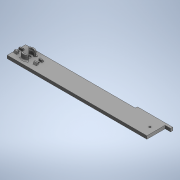
# Autodesk Inventor part: Arm Bottom Left
Saved by Autodesk Inventor 2020.5 (Build 245400000, 400)
## iProperties
Created: 2023-03-21
Part Number: Arm Bottom Left
Material: Generic
Document SubType Name: Modeling
Designer: Wes
Density: 1 g/cm^3
Appearance: Default
Author: Wes
Autodesk Inventor part; units mm, degrees
ref_plane "YZ Plane" through (0, 0, 0) normal (1, 0, 0) x (0, 1, 0)
ref_plane "XZ Plane" through (0, 0, 0) normal (0, 1, 0) x (-1, 0, 0)
ref_plane "XY Plane" through (0, 0, 0) normal (0, 0, 1) x (1, 0, 0)
sketch "Base" plane through (0, 0, 0) normal (0, 0, 1) x (1, 0, 0)
  line L0 (0, 0) -> (-30, 0)
  line L1 (-30, 0) -> (-30, 230)
  line L2 (-30, 230) -> (0, 230)
  line L3 (0, 230) -> (0, 0)
  dimension "d0" = 30
  dimension "d1" = 230
  constraints: 8 end point, 2 parallel, 1 horizontal, 1 perpendicular
  measures "d0" distance of L1.end L2.end
  measures "d1" distance of L0.end L1.end
extrude "Extrusion1" add sketch "Base" along normal blind 5
sketch "Axle Screw Countersink" plane through (0, 0, 5) normal (0, 0, 1) x (1, 0, 0)
  line L0 (-15, 0) -> (-15, 20) construction
  circle A0 centre (-15, 20) radius 3.15
  dimension "d4" = 20
  dimension "d58" = 6.3
  constraints: 2 end point, 1 centre point, 1 coincident, 1 vertical
  measures "d4" distance of L0.start L0.end
  measures "d58" diameter of A0
extrude "Extrusion2" cut sketch "Axle Screw Countersink" against normal blind 1.2
sketch "Motor Arm Center Fitting" plane through (0, 0, 5) normal (0, 0, 1) x (1, 0, 0)
  line L0 (-19.393, 15.95) -> (-19.393, 24.05) construction
  arc A0 (-19.393, 24.05) -> (-19.393, 15.95) centre (-15, 20) ccw
  line L1 (-19.393, 15.95) -> (-21.231, 14.2554)
  line L2 (-19.393, 24.05) -> (-21.231, 25.7446)
  line L3 (-15, 8.3504) -> (-15, 30.6989) construction
  arc A1 (-21.231, 25.7446) -> (-21.231, 14.2554) centre (-15, 20) ccw
  line L4 (-10.607, 15.95) -> (-10.607, 24.05) construction
  line L5 (-10.607, 15.95) -> (-19.393, 15.95) construction
  arc A2 (-10.607, 15.95) -> (-10.607, 24.05) centre (-15, 20) ccw
  line L6 (-10.607, 15.95) -> (-8.769, 14.2554)
  line L7 (-10.607, 24.05) -> (-8.769, 25.7446)
  arc A3 (-8.769, 14.2554) -> (-8.769, 25.7446) centre (-15, 20) ccw
  circle A4 centre (-15, 20) radius 5.975 construction
  point P0 (0, 0)
  point P1 (-15, 20)
  dimension "d18" = 11.95
  dimension "d19" = 8.1
  dimension "d20" = 8.1
  dimension "d21" = 2.5
  dimension "d22" = 2.5
  constraints: 16 end point, 12 point on circle, 5 centre point, 2 line through centre, 2 symmetric about line, 2 vertical, 1 concentric, 1 perpendicular, 2 other
  measures "d18" diameter of A4
  measures "d19" distance of L5.start L4.end
  measures "d20" distance of L5.end L0.end
  measures "d21" distance of L5.end L1.end
  measures "d22" distance of L0.end L2.end
extrude "Extrusion3" add sketch "Motor Arm Center Fitting" along normal blind 5
sketch "Motor Rotation Support" plane through (0, 0, 10) normal (0, 0, 1) x (1, 0, 0)
  line L0 (-20.975, 20) -> (-21.775, 20) construction
  circle A0 centre (-15, 20) radius 6.775 construction
  arc A1 (-19.9811, 24.5923) -> (-19.9811, 15.4077) centre (-15, 20) ccw
  line L1 (-21.775, 20) -> (-23.775, 20) construction
  circle A2 centre (-15, 20) radius 8.775 construction
  arc A3 (-21.4516, 25.9479) -> (-21.4516, 14.0521) centre (-15, 20) ccw
  line L2 (-21.4516, 14.0521) -> (-19.9811, 15.4077)
  line L3 (-19.9811, 24.5923) -> (-21.4516, 25.9479)
  line L4 (-15, 8.5295) -> (-15, 32.0479) construction
  line L5 (-8.5484, 14.0521) -> (-10.0189, 15.4077)
  arc A4 (-8.5484, 14.0521) -> (-8.5484, 25.9479) centre (-15, 20) ccw
  arc A5 (-10.0189, 15.4077) -> (-10.0189, 24.5923) centre (-15, 20) ccw
  line L6 (-10.0189, 24.5923) -> (-8.5484, 25.9479)
  point P0 (0, 0)
  point P1 (-21.231, 14.2554)
  point P2 (-21.231, 25.7446)
  dimension "d25" = 0.8
  dimension "d26" = 2
  constraints: 16 point on circle, 14 end point, 6 centre point, 4 symmetric about line, 2 coincident, 2 horizontal, 1 concentric, 1 vertical, 2 other
  measures "d25" distance of L0.start L0.end
  measures "d26" distance of L0.end L1.end
extrude "Extrusion4" add sketch "Motor Rotation Support" along normal blind 3.35
sketch "Motor Arm Screw Holes" plane through (0, 0, 5) normal (0, 0, 1) x (1, 0, 0)
  line L0 (-15, 20) -> (-15, 37.1) construction
  line L1 (-15, 20) -> (-15, 2.9) construction
  line L2 (-15, 20) -> (-15, 4.2) construction
  line L3 (-15, 20) -> (-15, 35.8) construction
  line L4 (-15, 4.2) -> (-15, 2.9) construction
  line L5 (-15, 35.8) -> (-15, 37.1) construction
  circle A0 centre (-15, 36.45) radius 1.175
  circle A1 centre (-15, 3.55) radius 1.175
  point P0 (0, 0)
  dimension "d59" = 34.2
  dimension "d60" = 31.6
  dimension "d61" = 2.35
  dimension "d62" = 2.35
  constraints: 12 end point, 3 vertical, 2 centre point, 2 midpoint, 2 point on line, 1 coincident, 1 collinear
  measures "d59" distance of L0.end L1.end
  measures "d60" distance of L3.end L2.end
  measures "d61" diameter of A0
  measures "d62" diameter of A1
extrude "Extrusion5" cut sketch "Motor Arm Screw Holes" against normal through all
sketch "Motor Arm Support" plane through (0, 0, 5) normal (0, 0, 1) x (1, 0, 0)
  line L0 (-15, 2.375) -> (-15, 6.875) construction
  line L1 (-15, 6.875) -> (-11.875, 6.875) construction
  line L2 (-15, 6.875) -> (-18.125, 6.875) construction
  line L3 (-21.0644, 20.2154) -> (-9.1144, 20.2154) construction
  line L4 (-15, 3.55) -> (-12.2, 3.55) construction
  line L5 (-15, 3.55) -> (-12.2, 3.55) construction
  line L6 (-15, 3.55) -> (-17.8, 3.55) construction
  line L7 (-15, 3.55) -> (-12.2, 3.55) construction
  line L8 (-18.125, 6.875) -> (-17.8, 3.55)
  line L9 (-17.8, 3.55) -> (-19.7905, 3.3554)
  line L10 (-19.7905, 3.3554) -> (-20.1155, 6.6804)
  line L11 (-20.1155, 6.6804) -> (-18.125, 6.875)
  line L12 (-11.875, 6.875) -> (-12.2, 3.55)
  line L13 (-12.2, 3.55) -> (-10.2095, 3.3554)
  line L14 (-9.8845, 6.6804) -> (-11.875, 6.875)
  line L15 (-10.2095, 3.3554) -> (-9.8845, 6.6804)
  line L16 (-17.8, 3.55) -> (-17.6054, 1.5595)
  line L17 (-17.6054, 1.5595) -> (-19.596, 1.3649)
  line L18 (-19.596, 1.3649) -> (-19.7905, 3.3554)
  line L19 (-12.2, 3.55) -> (-12.3946, 1.5595)
  line L20 (-12.3946, 1.5595) -> (-10.404, 1.3649)
  line L21 (-10.404, 1.3649) -> (-10.2095, 3.3554)
  line L22 (-17.8, 36.8809) -> (-19.7905, 37.0755)
  line L23 (-17.8, 36.8809) -> (-17.6054, 38.8714)
  line L24 (-17.6054, 38.8714) -> (-19.596, 39.066)
  line L25 (-19.596, 39.066) -> (-19.7905, 37.0755)
  line L26 (-18.125, 33.5559) -> (-17.8, 36.8809)
  line L27 (-19.7905, 37.0755) -> (-20.1155, 33.7505)
  line L28 (-20.1155, 33.7505) -> (-18.125, 33.5559)
  line L29 (-11.875, 33.5559) -> (-12.2, 36.8809)
  line L30 (-12.3946, 38.8714) -> (-10.404, 39.066)
  line L31 (-12.2, 36.8809) -> (-10.2095, 37.0755)
  line L32 (-10.404, 39.066) -> (-10.2095, 37.0755)
  line L33 (-10.2095, 37.0755) -> (-9.8845, 33.7505)
  line L34 (-9.8845, 33.7505) -> (-11.875, 33.5559)
  line L35 (-12.2, 36.8809) -> (-12.3946, 38.8714)
  point P0 (0, 0)
  dimension "d63" = 4.5
  dimension "d64" = 6.25
  dimension "d65" = 5.6
  dimension "d66" = 2
  dimension "d67" = 2
  constraints: 72 end point, 18 symmetric about line, 7 horizontal, 5 perpendicular, 2 collinear, 1 vertical
  measures "d63" distance of L0.start L1.start
  measures "d64" distance of L2.end L1.end
  measures "d65" distance of L8.end L4.end
  measures "d66" distance of L8.end L10.start
  measures "d67" distance of L8.end L17.start
extrude "Extrusion6" add sketch "Motor Arm Support" along normal blind 3
draft "FaceDraft1" angle 28 pull direction (0, 0, 1) faces at (-10.2309, 3.1368, 6) (-10.0577, 35.5223, 6) fixed edges at (-10.1443, 4.0227, 8) (-10.1443, 36.4082, 8)
draft "FaceDraft2" angle 28 pull direction (0, 0, 1) faces at (-19.7691, 37.2941, 6) (-19.9423, 4.9086, 6) fixed edges at (-19.8557, 36.4082, 8) (-19.8557, 4.0227, 8)
fillet "Fillet1" radius 2 4 edges at (-23.475, 20, 5) (-6.525, 20, 5) (-8.225, 20, 10) (-21.775, 20, 10)
sketch "Axle Hole" plane through (0, 0, 5) normal (0, 0, 1) x (1, 0, 0)
  line L0 (0, 230) -> (-30, 230) construction
  line L1 (-15, 230) -> (-15, 220) construction
  circle A0 centre (-15, 220) radius 1.5
  point P0 (0, 0)
  dimension "d73" = 10
  dimension "d74" = 3
  constraints: 2 end point, 1 centre point, 1 coincident, 1 midpoint, 1 vertical
  measures "d73" distance of L1.start L1.end
  measures "d74" diameter of A0
extrude "Extrusion7" cut sketch "Axle Hole" against normal through all
sketch "Sketch8" plane through (0, 0, 0) normal (0, 0, -1) x (-1, 0, 0)
  circle A0 centre (15, 220) radius 1.5 construction
  line L0 (15, 220) -> (15, 181) construction
  line L1 (15, 220) -> (15, 239) construction
  line L2 (30, 239) -> (33.5, 239)
  line L3 (33.5, 239) -> (33.5, 181)
  line L4 (33.5, 181) -> (30, 181)
  line L5 (30, 181) -> (30, 239)
  point P0 (0, 0)
  dimension "d77" = 39
  dimension "d78" = 19
  dimension "d79" = 3.5
  constraints: 12 end point, 2 parallel, 2 vertical, 1 horizontal, 1 perpendicular
  measures "d77" distance of L0.start L0.end
  measures "d78" distance of L0.start L1.end
  measures "d79" distance of L3.end L4.end
extrude "Extrusion8" add sketch "Sketch8" against normal up to surface (5 mm away)
body "Solid1"
